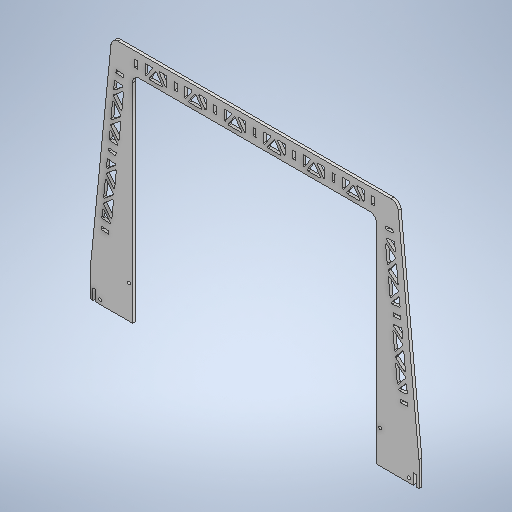
# Autodesk Inventor part: GateBrigeSide
Saved by Autodesk Inventor 2025.1 (Build 291241000, 241)
## iProperties
Created: 2025-03-30
Part Number: GateBrigeSide
Material: Všeobecné
Document SubType Name: Modeling
Designer: 42060
Density: 1 g/cm^3
Appearance: Výchozí
Author: 42060
Autodesk Inventor part; units mm, degrees
ref_plane "YZ Plane" through (0, 0, 0) normal (1, 0, 0) x (0, 1, 0)
ref_plane "XZ Plane" through (0, 0, 0) normal (0, 1, 0) x (-1, 0, 0)
ref_plane "XY Plane" through (0, 0, 0) normal (0, 0, 1) x (1, 0, 0)
sketch "Náčrt1" plane through (0, 0, 0) normal (0, 0, 1) x (1, 0, 0)
  line L0 (0, 0) -> (-160, 0)
  line L1 (-170, -10) -> (-170, -300)
  line L2 (-229, -300) -> (-229, -265.3)
  line L3 (-190.0509, 30) -> (0, 30)
  line L4 (0, 30) -> (0, 0)
  line L5 (-203.7, -249) -> (-170, -249)
  line L6 (-170, -249) -> (-170, -299)
  line L7 (-170, -299) -> (-220, -299)
  line L8 (-220, -299) -> (-220, -265.3)
  line L9 (-220, -265.3) -> (-203.7, -249)
  line L10 (-220, -299) -> (-170, -249) construction
  circle A0 centre (-215, -294) radius 2.1
  circle A1 centre (-175, -254) radius 2.1
  arc A2 (-160, 0) -> (-170, -10) centre (-160, -10) ccw
  line L11 (-200, 21.0077) -> (-229, -265.3)
  arc A3 (-190.0509, 30) -> (-200, 21.0077) centre (-190.0509, 20) ccw
  line L12 (-225, -300) -> (-225, -285)
  line L13 (-225, -285) -> (-221, -285)
  line L14 (-221, -285) -> (-221, -300)
  line L15 (-170, -300) -> (-221, -300)
  line L16 (-225, -300) -> (-229, -300)
  line L17 (-2, 10) -> (2, 10)
  line L18 (2, 10) -> (2, 20)
  line L19 (2, 20) -> (-2, 20)
  line L20 (-2, 20) -> (-2, 10)
  line L21 (-57, 20) -> (-57, 10)
  line L22 (-53, 20) -> (-57, 20)
  line L23 (-53, 10) -> (-53, 20)
  line L24 (-57, 10) -> (-53, 10)
  line L25 (-112, 20) -> (-112, 10)
  line L26 (-108, 20) -> (-112, 20)
  line L27 (-108, 10) -> (-108, 20)
  line L28 (-112, 10) -> (-108, 10)
  line L29 (-167, 20) -> (-167, 10)
  line L30 (-163, 20) -> (-167, 20)
  line L31 (-163, 10) -> (-163, 20)
  line L32 (-167, 10) -> (-163, 10)
  line L33 (-192.6355, -5.5165) -> (-182.6864, -6.5242)
  line L34 (-182.6864, -6.5242) -> (-183.0895, -10.5039)
  line L35 (-183.0895, -10.5039) -> (-193.0386, -9.4961)
  line L36 (-193.0386, -9.4961) -> (-192.6355, -5.5165)
  line L37 (-193.1669, -109.9948) -> (-203.116, -108.9871)
  line L38 (-192.7638, -106.0152) -> (-193.1669, -109.9948)
  line L39 (-203.116, -108.9871) -> (-202.7129, -105.0074)
  line L40 (-202.7129, -105.0074) -> (-192.7638, -106.0152)
  line L41 (-203.2443, -209.4857) -> (-213.1934, -208.478)
  line L42 (-202.8412, -205.5061) -> (-203.2443, -209.4857)
  line L43 (-213.1934, -208.478) -> (-212.7903, -204.4984)
  line L44 (-212.7903, -204.4984) -> (-202.8412, -205.5061)
  line L45 (0, 0) -> (160, 0)
  line L46 (170, -10) -> (170, -300)
  line L47 (229, -300) -> (229, -265.3)
  line L48 (190.0509, 30) -> (0, 30)
  line L49 (203.7, -249) -> (170, -249)
  line L50 (170, -249) -> (170, -299)
  line L51 (170, -299) -> (220, -299)
  line L52 (220, -299) -> (220, -265.3)
  line L53 (220, -265.3) -> (203.7, -249)
  line L54 (220, -299) -> (170, -249) construction
  circle A4 centre (215, -294) radius 2.1
  circle A5 centre (175, -254) radius 2.1
  arc A6 (170, -10) -> (160, 0) centre (160, -10) ccw
  line L55 (200, 21.0077) -> (229, -265.3)
  arc A7 (200, 21.0077) -> (190.0509, 30) centre (190.0509, 20) ccw
  line L56 (225, -300) -> (225, -285)
  line L57 (225, -285) -> (221, -285)
  line L58 (221, -285) -> (221, -300)
  line L59 (170, -300) -> (221, -300)
  line L60 (225, -300) -> (229, -300)
  line L61 (2, 10) -> (-2, 10)
  line L62 (-2, 10) -> (-2, 20)
  line L63 (-2, 20) -> (2, 20)
  line L64 (2, 20) -> (2, 10)
  line L65 (57, 20) -> (57, 10)
  line L66 (53, 20) -> (57, 20)
  line L67 (53, 10) -> (53, 20)
  line L68 (57, 10) -> (53, 10)
  line L69 (112, 20) -> (112, 10)
  line L70 (108, 20) -> (112, 20)
  line L71 (108, 10) -> (108, 20)
  line L72 (112, 10) -> (108, 10)
  line L73 (167, 20) -> (167, 10)
  line L74 (163, 20) -> (167, 20)
  line L75 (163, 10) -> (163, 20)
  line L76 (167, 10) -> (163, 10)
  line L77 (192.6355, -5.5165) -> (182.6864, -6.5242)
  line L78 (182.6864, -6.5242) -> (183.0895, -10.5039)
  line L79 (183.0895, -10.5039) -> (193.0386, -9.4961)
  line L80 (193.0386, -9.4961) -> (192.6355, -5.5165)
  line L81 (193.1669, -109.9948) -> (203.116, -108.9871)
  line L82 (192.7638, -106.0152) -> (193.1669, -109.9948)
  line L83 (203.116, -108.9871) -> (202.7129, -105.0074)
  line L84 (202.7129, -105.0074) -> (192.7638, -106.0152)
  line L85 (203.2443, -209.4857) -> (213.1934, -208.478)
  line L86 (202.8412, -205.5061) -> (203.2443, -209.4857)
  line L87 (213.1934, -208.478) -> (212.7903, -204.4984)
  line L88 (212.7903, -204.4984) -> (202.8412, -205.5061)
  line L89 (-36.6095, 7.1947) -> (-28.3278, 19.4124)
  line L90 (-26.6722, 19.4124) -> (-18.3905, 7.1947)
  line L91 (-19.2183, 5.6336) -> (-35.7817, 5.6336)
  line L92 (-22.6095, 20.5478) -> (-14.3278, 8.33)
  line L93 (-12.5, 8.8911) -> (-12.5, 21.1089)
  line L94 (-13.5, 22.1089) -> (-21.7817, 22.1089)
  line L95 (-32.3905, 20.5478) -> (-40.6722, 8.33)
  line L96 (-42.5, 8.8911) -> (-42.5, 21.1089)
  line L97 (-41.5, 22.1089) -> (-33.2183, 22.1089)
  line L98 (-53, 15) -> (-2, 15) construction
  arc A8 (-41.5, 22.1089) -> (-42.5, 21.1089) centre (-41.5, 21.1089) ccw
  arc A9 (-32.3905, 20.5478) -> (-33.2183, 22.1089) centre (-33.2183, 21.1089) ccw
  arc A10 (-42.5, 8.8911) -> (-40.6722, 8.33) centre (-41.5, 8.8911) ccw
  arc A11 (-36.6095, 7.1947) -> (-35.7817, 5.6336) centre (-35.7817, 6.6336) ccw
  arc A12 (-19.2183, 5.6336) -> (-18.3905, 7.1947) centre (-19.2183, 6.6336) ccw
  arc A13 (-26.6722, 19.4124) -> (-28.3278, 19.4124) centre (-27.5, 18.8514) ccw
  arc A14 (-21.7817, 22.1089) -> (-22.6095, 20.5478) centre (-21.7817, 21.1089) ccw
  arc A15 (-12.5, 21.1089) -> (-13.5, 22.1089) centre (-13.5, 21.1089) ccw
  arc A16 (-14.3278, 8.33) -> (-12.5, 8.8911) centre (-13.5, 8.8911) ccw
  arc A17 (-81.6722, 19.4124) -> (-83.3278, 19.4124) centre (-82.5, 18.8514) ccw
  line L99 (-91.6095, 7.1947) -> (-83.3278, 19.4124)
  line L100 (-68.5, 22.1089) -> (-76.7817, 22.1089)
  arc A18 (-67.5, 21.1089) -> (-68.5, 22.1089) centre (-68.5, 21.1089) ccw
  line L101 (-81.6722, 19.4124) -> (-73.3905, 7.1947)
  arc A19 (-74.2183, 5.6336) -> (-73.3905, 7.1947) centre (-74.2183, 6.6336) ccw
  line L102 (-77.6095, 20.5478) -> (-69.3278, 8.33)
  line L103 (-74.2183, 5.6336) -> (-90.7817, 5.6336)
  arc A20 (-69.3278, 8.33) -> (-67.5, 8.8911) centre (-68.5, 8.8911) ccw
  line L104 (-108, 15) -> (-57, 15) construction
  arc A21 (-96.5, 22.1089) -> (-97.5, 21.1089) centre (-96.5, 21.1089) ccw
  arc A22 (-97.5, 8.8911) -> (-95.6722, 8.33) centre (-96.5, 8.8911) ccw
  arc A23 (-91.6095, 7.1947) -> (-90.7817, 5.6336) centre (-90.7817, 6.6336) ccw
  arc A24 (-87.3905, 20.5478) -> (-88.2183, 22.1089) centre (-88.2183, 21.1089) ccw
  line L105 (-67.5, 8.8911) -> (-67.5, 21.1089)
  arc A25 (-76.7817, 22.1089) -> (-77.6095, 20.5478) centre (-76.7817, 21.1089) ccw
  line L106 (-96.5, 22.1089) -> (-88.2183, 22.1089)
  line L107 (-87.3905, 20.5478) -> (-95.6722, 8.33)
  line L108 (-97.5, 8.8911) -> (-97.5, 21.1089)
  arc A26 (-136.6722, 19.4124) -> (-138.3278, 19.4124) centre (-137.5, 18.8514) ccw
  line L109 (-146.6095, 7.1947) -> (-138.3278, 19.4124)
  line L110 (-123.5, 22.1089) -> (-131.7817, 22.1089)
  arc A27 (-122.5, 21.1089) -> (-123.5, 22.1089) centre (-123.5, 21.1089) ccw
  line L111 (-136.6722, 19.4124) -> (-128.3905, 7.1947)
  arc A28 (-129.2183, 5.6336) -> (-128.3905, 7.1947) centre (-129.2183, 6.6336) ccw
  line L112 (-132.6095, 20.5478) -> (-124.3278, 8.33)
  line L113 (-129.2183, 5.6336) -> (-145.7817, 5.6336)
  arc A29 (-124.3278, 8.33) -> (-122.5, 8.8911) centre (-123.5, 8.8911) ccw
  line L114 (-163, 15) -> (-112, 15) construction
  arc A30 (-151.5, 22.1089) -> (-152.5, 21.1089) centre (-151.5, 21.1089) ccw
  arc A31 (-152.5, 8.8911) -> (-150.6722, 8.33) centre (-151.5, 8.8911) ccw
  arc A32 (-146.6095, 7.1947) -> (-145.7817, 5.6336) centre (-145.7817, 6.6336) ccw
  arc A33 (-142.3905, 20.5478) -> (-143.2183, 22.1089) centre (-143.2183, 21.1089) ccw
  line L115 (-122.5, 8.8911) -> (-122.5, 21.1089)
  arc A34 (-131.7817, 22.1089) -> (-132.6095, 20.5478) centre (-131.7817, 21.1089) ccw
  line L116 (-151.5, 22.1089) -> (-143.2183, 22.1089)
  line L117 (-142.3905, 20.5478) -> (-150.6722, 8.33)
  line L118 (-152.5, 8.8911) -> (-152.5, 21.1089)
  line L119 (-194.0109, -19.4488) -> (-184.1326, -20.4494)
  line L120 (-183.6011, -22.2191) -> (-194.48, -31.0969)
  line L121 (-196.1072, -30.2213) -> (-195.1066, -20.3429)
  line L122 (-182.544, -28.7227) -> (-184.7467, -50.4692)
  line L123 (-186.5164, -51.0007) -> (-196.2883, -39.0261)
  line L124 (-196.1458, -37.6191) -> (-184.1711, -27.8471)
  line L125 (-195.9642, -45.7498) -> (-186.1923, -57.7245)
  line L126 (-186.3348, -59.1315) -> (-198.3095, -68.9034)
  line L127 (-199.9366, -68.0279) -> (-197.7339, -46.2813)
  line L128 (-188.0006, -65.6537) -> (-199.9752, -75.4256)
  line L129 (-200.1177, -76.8326) -> (-190.3458, -88.8073)
  line L130 (-188.5761, -88.2758) -> (-186.3734, -66.5292)
  line L131 (-199.7937, -83.5564) -> (-190.9158, -94.4353)
  line L132 (-191.7914, -96.0625) -> (-201.6698, -95.0619)
  line L133 (-202.5639, -93.9662) -> (-201.5633, -84.0878)
  line L134 (-189.0718, -19.9491) -> (-188.064, -10) construction
  arc A35 (-194.0109, -19.4488) -> (-195.1066, -20.3429) centre (-194.1117, -20.4437) ccw
  arc A36 (-183.6011, -22.2191) -> (-184.1326, -20.4494) centre (-184.2333, -21.4443) ccw
  arc A37 (-196.1072, -30.2213) -> (-194.48, -31.0969) centre (-195.1123, -30.3221) ccw
  arc A38 (-196.1458, -37.6191) -> (-196.2883, -39.0261) centre (-195.5135, -38.3938) ccw
  arc A39 (-186.5164, -51.0007) -> (-184.7467, -50.4692) centre (-185.7416, -50.3685) ccw
  arc A40 (-182.544, -28.7227) -> (-184.1711, -27.8471) centre (-183.5389, -28.6219) ccw
  arc A41 (-195.9642, -45.7498) -> (-197.7339, -46.2813) centre (-196.739, -46.3821) ccw
  arc A42 (-186.3348, -59.1315) -> (-186.1923, -57.7245) centre (-186.9671, -58.3567) ccw
  arc A43 (-199.9366, -68.0279) -> (-198.3095, -68.9034) centre (-198.9417, -68.1287) ccw
  arc A44 (-199.9752, -75.4256) -> (-200.1177, -76.8326) centre (-199.343, -76.2004) ccw
  arc A45 (-190.3458, -88.8073) -> (-188.5761, -88.2758) centre (-189.571, -88.175) ccw
  arc A46 (-186.3734, -66.5292) -> (-188.0006, -65.6537) centre (-187.3683, -66.4284) ccw
  arc A47 (-199.7937, -83.5564) -> (-201.5633, -84.0878) centre (-200.5684, -84.1886) ccw
  arc A48 (-202.5639, -93.9662) -> (-201.6698, -95.0619) centre (-201.569, -94.067) ccw
  arc A49 (-191.7914, -96.0625) -> (-190.9158, -94.4353) centre (-191.6906, -95.0676) ccw
  arc A50 (-212.6413, -193.4572) -> (-211.7472, -194.5528) centre (-211.6464, -193.5579) ccw
  line L135 (-201.8688, -195.5534) -> (-211.7472, -194.5528)
  arc A51 (-201.8688, -195.5534) -> (-200.9932, -193.9263) centre (-201.768, -194.5585) ccw
  arc A52 (-200.4232, -188.2982) -> (-198.6535, -187.7667) centre (-199.6484, -187.666) ccw
  line L136 (-209.871, -183.0473) -> (-200.9932, -193.9263)
  line L137 (-212.6413, -193.4572) -> (-211.6407, -183.5788)
  arc A53 (-209.871, -183.0473) -> (-211.6407, -183.5788) centre (-210.6458, -183.6796) ccw
  line L138 (-198.078, -165.1446) -> (-210.0526, -174.9165)
  line L139 (-210.1951, -176.3236) -> (-200.4232, -188.2982)
  line L140 (-198.6535, -187.7667) -> (-196.4508, -166.0201)
  arc A54 (-210.0526, -174.9165) -> (-210.1951, -176.3236) centre (-209.4204, -175.6913) ccw
  arc A55 (-210.014, -167.5188) -> (-208.3869, -168.3944) centre (-209.0191, -167.6196) ccw
  arc A56 (-196.4508, -166.0201) -> (-198.078, -165.1446) centre (-197.4457, -165.9194) ccw
  line L141 (-206.0416, -145.2407) -> (-196.2697, -157.2154)
  arc A57 (-196.4122, -158.6224) -> (-196.2697, -157.2154) centre (-197.0445, -157.8476) ccw
  line L142 (-210.014, -167.5188) -> (-207.8113, -145.7722)
  line L143 (-196.4122, -158.6224) -> (-208.3869, -168.3944)
  arc A58 (-196.5938, -150.4917) -> (-194.8241, -149.9602) centre (-195.819, -149.8594) ccw
  arc A59 (-206.0416, -145.2407) -> (-207.8113, -145.7722) centre (-206.8164, -145.873) ccw
  line L144 (-196.5938, -150.4917) -> (-206.3657, -138.517)
  arc A60 (-206.2232, -137.11) -> (-206.3657, -138.517) centre (-205.5909, -137.8848) ccw
  arc A61 (-206.1846, -129.7123) -> (-204.5574, -130.5878) centre (-205.1897, -129.813) ccw
  line L145 (-192.6214, -128.2136) -> (-194.8241, -149.9602)
  line L146 (-206.2232, -137.11) -> (-194.2485, -127.338)
  arc A62 (-192.6214, -128.2136) -> (-194.2485, -127.338) centre (-193.6163, -128.1128) ccw
  arc A63 (-193.6785, -121.71) -> (-194.21, -119.9403) centre (-194.3107, -120.9352) ccw
  line L147 (-199.1491, -119.44) -> (-198.1414, -109.4909) construction
  line L148 (-204.0883, -118.9397) -> (-194.21, -119.9403)
  arc A64 (-204.0883, -118.9397) -> (-205.184, -119.8339) centre (-204.1891, -119.9346) ccw
  line L149 (-193.6785, -121.71) -> (-204.5574, -130.5878)
  line L150 (-206.1846, -129.7123) -> (-205.184, -119.8339)
  line L151 (36.6095, 7.1947) -> (28.3278, 19.4124)
  line L152 (26.6722, 19.4124) -> (18.3905, 7.1947)
  line L153 (19.2183, 5.6336) -> (35.7817, 5.6336)
  line L154 (22.6095, 20.5478) -> (14.3278, 8.33)
  line L155 (12.5, 8.8911) -> (12.5, 21.1089)
  line L156 (13.5, 22.1089) -> (21.7817, 22.1089)
  line L157 (32.3905, 20.5478) -> (40.6722, 8.33)
  line L158 (42.5, 8.8911) -> (42.5, 21.1089)
  line L159 (41.5, 22.1089) -> (33.2183, 22.1089)
  line L160 (53, 15) -> (2, 15) construction
  arc A65 (42.5, 21.1089) -> (41.5, 22.1089) centre (41.5, 21.1089) ccw
  arc A66 (33.2183, 22.1089) -> (32.3905, 20.5478) centre (33.2183, 21.1089) ccw
  arc A67 (40.6722, 8.33) -> (42.5, 8.8911) centre (41.5, 8.8911) ccw
  arc A68 (35.7817, 5.6336) -> (36.6095, 7.1947) centre (35.7817, 6.6336) ccw
  arc A69 (18.3905, 7.1947) -> (19.2183, 5.6336) centre (19.2183, 6.6336) ccw
  arc A70 (28.3278, 19.4124) -> (26.6722, 19.4124) centre (27.5, 18.8514) ccw
  arc A71 (22.6095, 20.5478) -> (21.7817, 22.1089) centre (21.7817, 21.1089) ccw
  arc A72 (13.5, 22.1089) -> (12.5, 21.1089) centre (13.5, 21.1089) ccw
  arc A73 (12.5, 8.8911) -> (14.3278, 8.33) centre (13.5, 8.8911) ccw
  line L161 (67.5, 8.8911) -> (67.5, 21.1089)
  line L162 (96.5, 22.1089) -> (88.2183, 22.1089)
  arc A74 (97.5, 21.1089) -> (96.5, 22.1089) centre (96.5, 21.1089) ccw
  line L163 (97.5, 8.8911) -> (97.5, 21.1089)
  arc A75 (95.6722, 8.33) -> (97.5, 8.8911) centre (96.5, 8.8911) ccw
  arc A76 (67.5, 8.8911) -> (69.3278, 8.33) centre (68.5, 8.8911) ccw
  arc A77 (68.5, 22.1089) -> (67.5, 21.1089) centre (68.5, 21.1089) ccw
  arc A78 (88.2183, 22.1089) -> (87.3905, 20.5478) centre (88.2183, 21.1089) ccw
  arc A79 (83.3278, 19.4124) -> (81.6722, 19.4124) centre (82.5, 18.8514) ccw
  line L164 (87.3905, 20.5478) -> (95.6722, 8.33)
  line L165 (91.6095, 7.1947) -> (83.3278, 19.4124)
  arc A80 (77.6095, 20.5478) -> (76.7817, 22.1089) centre (76.7817, 21.1089) ccw
  arc A81 (90.7817, 5.6336) -> (91.6095, 7.1947) centre (90.7817, 6.6336) ccw
  line L166 (108, 15) -> (57, 15) construction
  line L167 (68.5, 22.1089) -> (76.7817, 22.1089)
  line L168 (77.6095, 20.5478) -> (69.3278, 8.33)
  line L169 (81.6722, 19.4124) -> (73.3905, 7.1947)
  arc A82 (73.3905, 7.1947) -> (74.2183, 5.6336) centre (74.2183, 6.6336) ccw
  line L170 (74.2183, 5.6336) -> (90.7817, 5.6336)
  line L171 (122.5, 8.8911) -> (122.5, 21.1089)
  line L172 (151.5, 22.1089) -> (143.2183, 22.1089)
  arc A83 (152.5, 21.1089) -> (151.5, 22.1089) centre (151.5, 21.1089) ccw
  line L173 (152.5, 8.8911) -> (152.5, 21.1089)
  arc A84 (150.6722, 8.33) -> (152.5, 8.8911) centre (151.5, 8.8911) ccw
  arc A85 (122.5, 8.8911) -> (124.3278, 8.33) centre (123.5, 8.8911) ccw
  arc A86 (123.5, 22.1089) -> (122.5, 21.1089) centre (123.5, 21.1089) ccw
  arc A87 (143.2183, 22.1089) -> (142.3905, 20.5478) centre (143.2183, 21.1089) ccw
  arc A88 (138.3278, 19.4124) -> (136.6722, 19.4124) centre (137.5, 18.8514) ccw
  line L174 (142.3905, 20.5478) -> (150.6722, 8.33)
  line L175 (146.6095, 7.1947) -> (138.3278, 19.4124)
  arc A89 (132.6095, 20.5478) -> (131.7817, 22.1089) centre (131.7817, 21.1089) ccw
  arc A90 (145.7817, 5.6336) -> (146.6095, 7.1947) centre (145.7817, 6.6336) ccw
  line L176 (163, 15) -> (112, 15) construction
  line L177 (123.5, 22.1089) -> (131.7817, 22.1089)
  line L178 (132.6095, 20.5478) -> (124.3278, 8.33)
  line L179 (136.6722, 19.4124) -> (128.3905, 7.1947)
  arc A91 (128.3905, 7.1947) -> (129.2183, 5.6336) centre (129.2183, 6.6336) ccw
  line L180 (129.2183, 5.6336) -> (145.7817, 5.6336)
  line L181 (194.0109, -19.4488) -> (184.1326, -20.4494)
  line L182 (183.6011, -22.2191) -> (194.48, -31.0969)
  line L183 (196.1072, -30.2213) -> (195.1066, -20.3429)
  line L184 (182.544, -28.7227) -> (184.7467, -50.4692)
  line L185 (186.5164, -51.0007) -> (196.2883, -39.0261)
  line L186 (196.1458, -37.6191) -> (184.1711, -27.8471)
  line L187 (195.9642, -45.7498) -> (186.1923, -57.7245)
  line L188 (186.3348, -59.1315) -> (198.3095, -68.9034)
  line L189 (199.9366, -68.0279) -> (197.7339, -46.2813)
  line L190 (188.0006, -65.6537) -> (199.9752, -75.4256)
  line L191 (200.1177, -76.8326) -> (190.3458, -88.8073)
  line L192 (188.5761, -88.2758) -> (186.3734, -66.5292)
  line L193 (199.7937, -83.5564) -> (190.9158, -94.4353)
  line L194 (191.7914, -96.0625) -> (201.6698, -95.0619)
  line L195 (202.5639, -93.9662) -> (201.5633, -84.0878)
  line L196 (189.0718, -19.9491) -> (188.064, -10) construction
  arc A92 (195.1066, -20.3429) -> (194.0109, -19.4488) centre (194.1117, -20.4437) ccw
  arc A93 (184.1326, -20.4494) -> (183.6011, -22.2191) centre (184.2333, -21.4443) ccw
  arc A94 (194.48, -31.0969) -> (196.1072, -30.2213) centre (195.1123, -30.3221) ccw
  arc A95 (196.2883, -39.0261) -> (196.1458, -37.6191) centre (195.5135, -38.3938) ccw
  arc A96 (184.7467, -50.4692) -> (186.5164, -51.0007) centre (185.7416, -50.3685) ccw
  arc A97 (184.1711, -27.8471) -> (182.544, -28.7227) centre (183.5389, -28.6219) ccw
  arc A98 (197.7339, -46.2813) -> (195.9642, -45.7498) centre (196.739, -46.3821) ccw
  arc A99 (186.1923, -57.7245) -> (186.3348, -59.1315) centre (186.9671, -58.3567) ccw
  arc A100 (198.3095, -68.9034) -> (199.9366, -68.0279) centre (198.9417, -68.1287) ccw
  arc A101 (200.1177, -76.8326) -> (199.9752, -75.4256) centre (199.343, -76.2004) ccw
  arc A102 (188.5761, -88.2758) -> (190.3458, -88.8073) centre (189.571, -88.175) ccw
  arc A103 (188.0006, -65.6537) -> (186.3734, -66.5292) centre (187.3683, -66.4284) ccw
  arc A104 (201.5633, -84.0878) -> (199.7937, -83.5564) centre (200.5684, -84.1886) ccw
  arc A105 (201.6698, -95.0619) -> (202.5639, -93.9662) centre (201.569, -94.067) ccw
  arc A106 (190.9158, -94.4353) -> (191.7914, -96.0625) centre (191.6906, -95.0676) ccw
  arc A107 (194.21, -119.9403) -> (193.6785, -121.71) centre (194.3107, -120.9352) ccw
  arc A108 (194.2485, -127.338) -> (192.6214, -128.2136) centre (193.6163, -128.1128) ccw
  line L197 (204.0883, -118.9397) -> (194.21, -119.9403)
  line L198 (193.6785, -121.71) -> (204.5574, -130.5878)
  line L199 (206.1846, -129.7123) -> (205.184, -119.8339)
  line L200 (206.2232, -137.11) -> (194.2485, -127.338)
  arc A109 (205.184, -119.8339) -> (204.0883, -118.9397) centre (204.1891, -119.9346) ccw
  arc A110 (204.5574, -130.5878) -> (206.1846, -129.7123) centre (205.1897, -129.813) ccw
  line L201 (192.6214, -128.2136) -> (194.8241, -149.9602)
  arc A111 (207.8113, -145.7722) -> (206.0416, -145.2407) centre (206.8164, -145.873) ccw
  line L202 (196.5938, -150.4917) -> (206.3657, -138.517)
  arc A112 (206.3657, -138.517) -> (206.2232, -137.11) centre (205.5909, -137.8848) ccw
  arc A113 (194.8241, -149.9602) -> (196.5938, -150.4917) centre (195.819, -149.8594) ccw
  line L203 (206.0416, -145.2407) -> (196.2697, -157.2154)
  arc A114 (196.2697, -157.2154) -> (196.4122, -158.6224) centre (197.0445, -157.8476) ccw
  arc A115 (198.078, -165.1446) -> (196.4508, -166.0201) centre (197.4457, -165.9194) ccw
  line L204 (196.4122, -158.6224) -> (208.3869, -168.3944)
  arc A116 (208.3869, -168.3944) -> (210.014, -167.5188) centre (209.0191, -167.6196) ccw
  line L205 (210.014, -167.5188) -> (207.8113, -145.7722)
  arc A117 (200.9932, -193.9263) -> (201.8688, -195.5534) centre (201.768, -194.5585) ccw
  arc A118 (211.7472, -194.5528) -> (212.6413, -193.4572) centre (211.6464, -193.5579) ccw
  arc A119 (198.6535, -187.7667) -> (200.4232, -188.2982) centre (199.6484, -187.666) ccw
  line L206 (212.6413, -193.4572) -> (211.6407, -183.5788)
  line L207 (209.871, -183.0473) -> (200.9932, -193.9263)
  arc A120 (211.6407, -183.5788) -> (209.871, -183.0473) centre (210.6458, -183.6796) ccw
  line L208 (210.1951, -176.3236) -> (200.4232, -188.2982)
  arc A121 (210.1951, -176.3236) -> (210.0526, -174.9165) centre (209.4204, -175.6913) ccw
  line L209 (198.6535, -187.7667) -> (196.4508, -166.0201)
  line L210 (198.078, -165.1446) -> (210.0526, -174.9165)
  line L211 (201.8688, -195.5534) -> (211.7472, -194.5528)
  point P0 (2, 15)
  point P1 (0, 15)
  point P2 (0, 10)
  point P3 (-55, 10)
  point P4 (-110, 10)
  point P5 (-165, 10)
  point P6 (55, 10)
  point P7 (108, 15)
  point P8 (110, 10)
  point P9 (163, 15)
  point P10 (165, 10)
  point P11 (-27.5, 20.6336)
  point P12 (-12.5, 5.6336)
  point P13 (-31.3323, 22.1089)
  point P14 (-42.5, 22.1089)
  point P15 (-27.5, 5.6336)
  point P16 (-27.5, 15)
  point P17 (-12.5, 15)
  point P18 (-2, 15)
  point P19 (-82.5, 20.6336)
  point P20 (-82.5, 15)
  point P21 (-82.5, 5.6336)
  point P22 (-86.3323, 22.1089)
  point P23 (-97.5, 22.1089)
  point P24 (-67.5, 5.6336)
  point P25 (-67.5, 15)
  point P26 (-137.5, 20.6336)
  point P27 (-137.5, 15)
  point P28 (-137.5, 5.6336)
  point P29 (-141.3323, 22.1089)
  point P30 (-152.5, 22.1089)
  point P31 (-122.5, 5.6336)
  point P32 (-122.5, 15)
  point P33 (-195.0059, -19.348)
  point P34 (-181.7306, -20.6927)
  point P35 (-196.3505, -32.6233)
  point P36 (-182.3007, -26.3207)
  point P37 (-184.99, -52.8712)
  point P38 (-196.9206, -38.2513)
  point P39 (-197.4906, -43.8794)
  point P40 (-185.56, -58.4992)
  point P41 (-200.1799, -70.4298)
  point P42 (-186.1301, -64.1273)
  point P43 (-200.75, -76.0579)
  point P44 (-188.8194, -90.6777)
  point P45 (-201.32, -81.6859)
  point P46 (-189.3895, -96.3058)
  point P47 (-202.6647, -94.9611)
  point P48 (-212.7421, -194.4521)
  point P49 (-199.4669, -195.7967)
  point P50 (-198.8968, -190.1687)
  point P51 (-211.3974, -181.1769)
  point P52 (-210.8274, -175.5488)
  point P53 (-210.2573, -169.9207)
  point P54 (-196.2075, -163.6182)
  point P55 (-195.6374, -157.9902)
  point P56 (-195.0674, -152.3621)
  point P57 (-207.568, -143.3703)
  point P58 (-206.998, -137.7422)
  point P59 (-206.4279, -132.1142)
  point P60 (-192.3781, -125.8117)
  point P61 (-191.808, -120.1836)
  point P62 (-205.0833, -118.839)
  point P63 (27.5, 20.6336)
  point P64 (12.5, 5.6336)
  point P65 (31.3323, 22.1089)
  point P66 (42.5, 22.1089)
  point P67 (27.5, 5.6336)
  point P68 (27.5, 15)
  point P69 (12.5, 15)
  point P70 (67.5, 5.6336)
  point P71 (67.5, 15)
  point P72 (82.5, 20.6336)
  point P73 (86.3323, 22.1089)
  point P74 (97.5, 22.1089)
  point P75 (82.5, 15)
  point P76 (82.5, 5.6336)
  point P77 (122.5, 5.6336)
  point P78 (122.5, 15)
  point P79 (137.5, 20.6336)
  point P80 (141.3323, 22.1089)
  point P81 (152.5, 22.1089)
  point P82 (137.5, 15)
  point P83 (137.5, 5.6336)
  point P84 (195.0059, -19.348)
  point P85 (181.7306, -20.6927)
  point P86 (196.3505, -32.6233)
  point P87 (182.3007, -26.3207)
  point P88 (184.99, -52.8712)
  point P89 (196.9206, -38.2513)
  point P90 (197.4906, -43.8794)
  point P91 (185.56, -58.4992)
  point P92 (200.1799, -70.4298)
  point P93 (186.1301, -64.1273)
  point P94 (200.75, -76.0579)
  point P95 (188.8194, -90.6777)
  point P96 (201.32, -81.6859)
  point P97 (189.3895, -96.3058)
  point P98 (202.6647, -94.9611)
  point P99 (191.808, -120.1836)
  point P100 (192.3781, -125.8117)
  point P101 (199.1491, -119.44)
  point P102 (205.0833, -118.839)
  point P103 (206.4279, -132.1142)
  point P104 (206.998, -137.7422)
  point P105 (195.0674, -152.3621)
  point P106 (207.568, -143.3703)
  point P107 (195.6374, -157.9902)
  point P108 (196.2075, -163.6182)
  point P109 (210.2573, -169.9207)
  point P110 (212.7421, -194.4521)
  point P111 (199.4669, -195.7967)
  point P112 (198.8968, -190.1687)
  point P113 (210.8274, -175.5488)
  point P114 (211.3974, -181.1769)
  dimension "d0" = 50
  dimension "d1" = 50
  dimension "d3" = 33.7
  dimension "d4" = 45
  dimension "d5" = 0
  dimension "d6" = 4.2
  dimension "d7" = 5
  dimension "d8" = 5
  dimension "d10" = 170
  dimension "d12" = 30
  dimension "d14" = 10
  dimension "d16" = 15
  dimension "d17" = 1
  dimension "d18" = 4
  dimension "d19" = 1
  dimension "d20" = 4
  dimension "d21" = 300
  dimension "d22" = 30
  dimension "d25" = 4
  dimension "d26" = 10
  dimension "d29" = 55
  dimension "d34" = 4
  dimension "d35" = 10
  dimension "d36" = 10
  dimension "d39" = 100
  dimension "d46" = 4
  dimension "d47" = 4
  dimension "d50" = 15
  dimension "d51" = 30
  dimension "d52" = 1
  dimension "d55" = 55
  dimension "d60" = 10
  dimension "d61" = 10
  dimension "d63" = 4
  dimension "d64" = 4
  dimension "d65" = 4
  dimension "d66" = 4
  dimension "d67" = 1
  dimension "d70" = 100
  dimension "d77" = 55
  dimension "d84" = 100
  constraints: 424 end point, 236 point on circle, 210 point on line, 152 symmetric about line, 122 centre point, 52 tangent, 24 equal radius, 18 perpendicular, 17 parallel, 9 midpoint, 8 horizontal, 7 collinear, 5 horizontal alignment, 4 equal length, 3 vertical alignment, 1 vertical, 481 other
  measures "d0" distance of L5.end L6.end
  measures "d1" distance of L6.end L7.end
  measures "d3" distance of L5.start L5.end
  measures "d4" angle of L5 L9
  measures "d5" distance between parallel lines of L1 L6
  measures "d6" diameter of A1
  measures "d7" distance from line of L5 A1.centre
  measures "d8" distance from line of L7 A0.centre
  measures "d10" distance between parallel lines of L1 L4
  measures "d12" distance between parallel lines of L0 L3
  measures "d14" radius of A3
  measures "d16" distance between parallel lines of L16 L13
  measures "d17" distance between parallel lines of L7 L15
  measures "d18" distance between parallel lines of L14 L12
  measures "d19" distance between parallel lines of L8 L14
  measures "d20" distance between parallel lines of L12 L2
  measures "d21" distance between parallel lines of L15 L0
  measures "d22" distance from line of L11.start L1
  measures "d25" distance of L18.end L19.end
  measures "d26" distance of L17.end L18.end
  measures "d29" distance of L19.end L21.start
  measures "d34" distance of L35.end L33.start
  measures "d35" distance of L33.start L33.end
  measures "d36" distance between parallel lines of L11 L36
  measures "d39" distance of L34.end L37.start
  measures "d46" distance between parallel lines of L89 L95
  measures "d47" distance between parallel lines of L92 L90
  measures "d50" distance from line of L91 point (-27.5, 20.634)
  measures "d51" distance between parallel lines of L93 L96
  measures "d52" radius of A8
  measures "d55" distance of point (-27.5, 20.634) point (-82.5, 20.634)
  measures "d60" distance between parallel lines of L35 L119
  measures "d61" distance between parallel lines of L132 L40
  measures "d63" distance between parallel lines of L124 L120
  measures "d64" distance between parallel lines of L125 L123
  measures "d65" distance between parallel lines of L128 L126
  measures "d66" distance between parallel lines of L129 L131
  measures "d67" radius of A35
  measures "d70" distance of point (-202.665, -94.961) point (-212.742, -194.452)
  measures "d77" distance of point (12.5, 5.634) point (67.5, 5.634)
  measures "d84" distance of point (181.731, -20.693) point (191.808, -120.184)
extrude "Vysunutí1" add sketch "Náčrt1" along normal blind 4 contours L0 A2 L1 L5 L9 L8 L7 L15 L14 L13 L12 L16 L2 L11 A3 L3 L4 L19 L20 L17 | L4 L17 L18 L19 L48 A7 L55 L47 L60 L56 L57 L58 L59 L46 L51 L52 L53 L49 A6 L45 | L1 L7 L8 L9 L5 | L49 L53 L52 L51 L46
equation "\"d25\" = d18"
equation "\"d34\" = d18"
equation "\"d35\" = d26"
equation "\"d36\" = d26"
equation "\"d44\" = d18"
